Autodesk Inventor part; units mm, degrees
note: some values were not read from the file. Chosen so that the rebuilt part matches the saved one: direction of "Hole2".
(part 7 of 18)
  spline S53 degree 3 poles (-10045.5969, -10030.692) (-10045.5963, -10030.6873) (-10045.5949, -10030.677) (-10045.5853, -10030.6623) (-10045.5707, -10030.6477) (-10045.5504, -10030.6334) (-10045.5248, -10030.6195) (-10045.482, -10030.6008) (-10045.433, -10030.585) (-10045.3785, -10030.5714) (-10045.3141, -10030.5581) (-10045.2258, -10030.5447) (-10045.1146, -10030.5354) (-10045, -10030.532) (-10044.8854, -10030.5354) (-10044.7742, -10030.5447) (-10044.6859, -10030.5581) (-10044.6215, -10030.5714) (-10044.567, -10030.585) (-10044.518, -10030.6008) (-10044.4752, -10030.6195) (-10044.4496, -10030.6334) (-10044.4293, -10030.6477) (-10044.4147, -10030.6623) (-10044.4051, -10030.677) (-10044.4037, -10030.6873) (-10044.4031, -10030.692) knots 0 0 0 0 0.011067 0.024078 0.039928 0.05914 0.081934 0.10802 0.168059 0.202015 0.239296 0.321668 0.410563 0.5 0.589437 0.678332 0.760704 0.797985 0.831941 0.89198 0.918066 0.94086 0.960072 0.975922 0.988933 1 1 1 1
  spline S54 degree 3 poles (-10044.4031, -10030.692) (-10044.4037, -10030.6967) (-10044.405, -10030.7067) (-10044.4147, -10030.7206) (-10044.4293, -10030.7339) (-10044.4497, -10030.7464) (-10044.4753, -10030.758) (-10044.5182, -10030.7731) (-10044.5672, -10030.7852) (-10044.6216, -10030.7953) (-10044.6861, -10030.8049) (-10044.7744, -10030.8142) (-10044.8855, -10030.8205) (-10045, -10030.8227) (-10045.1145, -10030.8205) (-10045.2256, -10030.8142) (-10045.3139, -10030.8049) (-10045.3784, -10030.7953) (-10045.4328, -10030.7852) (-10045.4818, -10030.7731) (-10045.5247, -10030.758) (-10045.5503, -10030.7464) (-10045.5707, -10030.7339) (-10045.5853, -10030.7206) (-10045.595, -10030.7067) (-10045.5963, -10030.6967) (-10045.5969, -10030.692) knots 0 0 0 0 0.010997 0.023628 0.038954 0.057614 0.079908 0.105595 0.165209 0.199149 0.236543 0.319515 0.409403 0.5 0.590597 0.680485 0.763457 0.800851 0.834791 0.894405 0.920092 0.942386 0.961046 0.976372 0.989003 1 1 1 1
  spline S55 degree 3 poles (-10044.4031, -10007.502) (-10044.4037, -10007.5067) (-10044.4051, -10007.517) (-10044.4147, -10007.5317) (-10044.4293, -10007.5463) (-10044.4496, -10007.5606) (-10044.4752, -10007.5745) (-10044.518, -10007.5931) (-10044.567, -10007.6089) (-10044.6215, -10007.6226) (-10044.6859, -10007.6359) (-10044.7742, -10007.6492) (-10044.8854, -10007.6586) (-10045, -10007.6619) (-10045.1146, -10007.6586) (-10045.2258, -10007.6492) (-10045.3141, -10007.6359) (-10045.3785, -10007.6226) (-10045.433, -10007.6089) (-10045.482, -10007.5931) (-10045.5248, -10007.5745) (-10045.5504, -10007.5606) (-10045.5707, -10007.5463) (-10045.5853, -10007.5317) (-10045.5949, -10007.517) (-10045.5963, -10007.5067) (-10045.5969, -10007.502) knots 0 0 0 0 0.011067 0.024078 0.039928 0.05914 0.081934 0.10802 0.168059 0.202015 0.239296 0.321668 0.410563 0.5 0.589437 0.678332 0.760704 0.797985 0.831941 0.89198 0.918066 0.94086 0.960072 0.975922 0.988933 1 1 1 1
  spline S56 degree 3 poles (-10045.5969, -10007.502) (-10045.5963, -10007.4973) (-10045.595, -10007.4873) (-10045.5853, -10007.4734) (-10045.5707, -10007.4601) (-10045.5503, -10007.4476) (-10045.5247, -10007.436) (-10045.4818, -10007.4208) (-10045.4328, -10007.4087) (-10045.3784, -10007.3987) (-10045.3139, -10007.3891) (-10045.2256, -10007.3798) (-10045.1145, -10007.3735) (-10045, -10007.3713) (-10044.8855, -10007.3735) (-10044.7744, -10007.3798) (-10044.6861, -10007.3891) (-10044.6216, -10007.3987) (-10044.5672, -10007.4087) (-10044.5182, -10007.4208) (-10044.4753, -10007.436) (-10044.4497, -10007.4476) (-10044.4293, -10007.4601) (-10044.4147, -10007.4734) (-10044.405, -10007.4873) (-10044.4037, -10007.4973) (-10044.4031, -10007.502) knots 0 0 0 0 0.010997 0.023628 0.038954 0.057614 0.079908 0.105595 0.165209 0.199149 0.236543 0.319515 0.409403 0.5 0.590597 0.680485 0.763457 0.800851 0.834791 0.894405 0.920092 0.942386 0.961046 0.976372 0.989003 1 1 1 1
  line L1792 (-10042.592, -10023.3102) -> (-10042.5, -10023.3102)
  line L1793 (-10042.5, -10028.2512) -> (-10043.1, -10028.2512)
  line L1794 (-10042.5, -10023.3102) -> (-10042.5, -10028.2512)
  line L1795 (-10042.5, -10014.8837) -> (-10042.592, -10014.8837)
  line L1796 (-10042.5, -10009.9428) -> (-10042.5, -10014.8837)
  line L1797 (-10043.1, -10009.9428) -> (-10042.5, -10009.9428)
  line L1798 (-10043.1, -10023.097) -> (-10043.1, -10028.2512)
  line L1799 (-10043.1, -10009.9428) -> (-10043.1, -10015.097)
  line L1800 (-10042.5, -10007.147) -> (-10042.5, -10009.9428)
  line L1801 (-10042.5, -10028.2512) -> (-10042.5, -10031.047)
  line L1802 (-10047.5, -10015.097) -> (-10047.5, -10007.147)
  line L1803 (-10047.5, -10031.047) -> (-10047.5, -10023.097)
  line L1804 (-10042.5, -10031.047) -> (-10047.5, -10031.047)
  line L1805 (-10042.5, -10007.147) -> (-10047.5, -10007.147)
  line L1806 (-10042.5, -10014.8837) -> (-10042.5, -10015.1936)
  line L1807 (-10042.5, -10015.1936) -> (-10042.592, -10015.1936)
  line L1808 (-10042.5, -10015.1936) -> (-10042.5, -10023.3102)
  line L1809 (-10057.5, -10028.1794) -> (-10057.5, -10022.4221)
  line L1810 (-10057.5, -10015.7719) -> (-10057.5, -10010.0146)
  line L1811 (-10057.5, -10008.4468) -> (-10057.5, -10007.8837)
  line L1812 (-10057.5, -10030.3103) -> (-10057.5, -10029.7472)
  line L1813 (-10047.5, -10007.8837) -> (-10057.5, -10007.8837)
  line L1814 (-10057.5, -10030.3103) -> (-10047.5, -10030.3103)
  spline S57 degree 3 poles (-10050.101, -10027.8648) (-10050.2112, -10027.8645) (-10050.4351, -10027.8611) (-10050.7676, -10027.843) (-10051.0408, -10027.8129) (-10051.2301, -10027.7795) (-10051.3223, -10027.7451) (-10051.3848, -10027.7216) (-10051.3872, -10027.6724) (-10051.3472, -10027.6448) (-10051.2666, -10027.61) (-10051.0804, -10027.5729) (-10050.8071, -10027.5414) (-10050.4756, -10027.5234) (-10050.1423, -10027.519) (-10049.8093, -10027.5266) (-10049.4755, -10027.5466) (-10049.2034, -10027.5785) (-10049.0137, -10027.6143) (-10048.9225, -10027.6467) (-10048.8568, -10027.6705) (-10048.8566, -10027.7199) (-10048.8981, -10027.7462) (-10048.9787, -10027.777) (-10049.1645, -10027.8141) (-10049.4369, -10027.8433) (-10049.7691, -10027.8609) (-10049.9917, -10027.865) (-10050.101, -10027.8648) knots 0 0 0 0 0.063707 0.129495 0.191912 0.223688 0.23829 0.25135 0.256604 0.263018 0.277149 0.308538 0.37104 0.436878 0.500023 0.563695 0.629383 0.692836 0.723161 0.738573 0.75181 0.756962 0.76326 0.777952 0.808043 0.871314 0.936843 1 1 1 1
  spline S58 degree 3 poles (-10050.1826, -10030.061) (-10050.4053, -10030.0603) (-10050.7291, -10030.05) (-10051.1255, -10030.0499) (-10051.2836, -10030.0122) (-10051.3774, -10030.0214) (-10051.3875, -10029.9848) (-10051.307, -10029.9741) (-10051.2197, -10029.9555) (-10050.9994, -10029.9405) (-10050.7296, -10029.927) (-10050.3957, -10029.9197) (-10049.9493, -10029.9156) (-10049.5164, -10029.9313) (-10049.1193, -10029.9348) (-10048.9604, -10029.9745) (-10048.8659, -10029.9652) (-10048.8554, -10030.0025) (-10048.9378, -10030.0112) (-10049.0249, -10030.0292) (-10049.246, -10030.0414) (-10049.6233, -10030.0575) (-10049.9596, -10030.0616) (-10050.1826, -10030.061) knots 0 0 0 0 0.131392 0.195062 0.224866 0.236537 0.238771 0.243638 0.272647 0.302988 0.368078 0.435032 0.499113 0.631038 0.694715 0.724747 0.73665 0.738894 0.743873 0.773079 0.803452 0.868455 1 1 1 1
  spline S59 degree 3 poles (-10050.1826, -10010.6731) (-10050.2929, -10010.6727) (-10050.5175, -10010.6697) (-10050.8464, -10010.6478) (-10051.127, -10010.6184) (-10051.2936, -10010.571) (-10051.3855, -10010.5349) (-10051.3867, -10010.4859) (-10051.3246, -10010.4425) (-10051.2136, -10010.412) (-10051.0014, -10010.3752) (-10050.7253, -10010.348) (-10050.394, -10010.3316) (-10050.0607, -10010.3274) (-10049.7273, -10010.3345) (-10049.3981, -10010.354) (-10049.1186, -10010.3846) (-10048.951, -10010.4283) (-10048.8591, -10010.4605) (-10048.8553, -10010.51) (-10048.9209, -10010.5537) (-10049.03, -10010.5814) (-10049.2424, -10010.6228) (-10049.5173, -10010.6499) (-10049.8505, -10010.669) (-10050.0733, -10010.6734) (-10050.1826, -10010.6731) knots 0 0 0 0 0.063774 0.129476 0.191917 0.222516 0.235727 0.240982 0.247121 0.27643 0.308417 0.371002 0.43691 0.500019 0.563738 0.62925 0.691939 0.722123 0.735387 0.74054 0.746943 0.777028 0.807219 0.871188 0.93687 1 1 1 1
  line L1815 (-10057.5, -10010.0146) -> (-10057.5, -10008.4468)
  line L1816 (-10057.5, -10029.7472) -> (-10057.5, -10028.1794)
  spline S60 degree 3 poles (-10050.101, -10008.2758) (-10050.3249, -10008.2751) (-10050.6589, -10008.2732) (-10051.0379, -10008.2488) (-10051.2309, -10008.2402) (-10051.3162, -10008.2166) (-10051.382, -10008.2231) (-10051.3853, -10008.1857) (-10051.34, -10008.1823) (-10051.2677, -10008.1628) (-10051.076, -10008.154) (-10050.8073, -10008.1395) (-10050.475, -10008.134) (-10050.0295, -10008.1322) (-10049.5838, -10008.1356) (-10049.2069, -10008.1566) (-10049.0122, -10008.164) (-10048.9298, -10008.1856) (-10048.8582, -10008.1781) (-10048.8591, -10008.2157) (-10048.9046, -10008.2188) (-10048.9776, -10008.2383) (-10049.1684, -10008.2498) (-10049.5444, -10008.2725) (-10049.8785, -10008.2765) (-10050.101, -10008.2758) knots 0 0 0 0 0.132092 0.195475 0.227359 0.241584 0.252969 0.255186 0.260256 0.27356 0.304855 0.368241 0.435353 0.499807 0.631725 0.696074 0.726444 0.741485 0.752997 0.755195 0.760334 0.774394 0.8045 0.86873 1 1 1 1
  line L1817 (-10055.03, -10015.097) -> (-10062.35, -10017.097)
  line L1818 (-10062.35, -10021.097) -> (-10055.03, -10023.097)
  line L1819 (-10043.608, -10015.097) -> (-10055.03, -10015.097)
  line L1820 (-10043.608, -10023.097) -> (-10055.03, -10023.097)
  line L1821 (-10062.35, -10017.097) -> (-10062.35, -10021.097)
  line L1822 (-10043.608, -10015.097) -> (-10042.592, -10015.097)
  line L1823 (-10043.608, -10023.097) -> (-10042.592, -10023.097)
  line L1824 (-10042.592, -10015.097) -> (-10042.592, -10023.097)
  line L1825 (-10042.592, -10027.222) -> (-10042.592, -10027.3968)
  line L1826 (-10043.1, -10027.222) -> (-10042.592, -10027.222)
  line L1827 (-10042.592, -10023.5196) -> (-10042.592, -10027.222)
  line L1828 (-10042.592, -10023.5196) -> (-10042.592, -10023.097)
  line L1829 (-10042.592, -10015.097) -> (-10042.592, -10014.6744)
  line L1830 (-10042.592, -10010.972) -> (-10042.592, -10014.6744)
  line L1831 (-10043.1, -10010.972) -> (-10042.592, -10010.972)
  line L1832 (-10042.592, -10010.7972) -> (-10042.592, -10010.972)
  line L1833 (-10043.1, -10027.3968) -> (-10042.592, -10027.3968)
  line L1834 (-10043.1, -10010.7972) -> (-10042.592, -10010.7972)
  line L1835 (-10039.5, -10030.097) -> (-10039.5, -10008.097)
  line L1836 (-10006.5, -10030.097) -> (-10006.5, -10008.097)
  line L1837 (-10006.5, -10030.097) -> (-10039.5, -10030.097)
  line L1838 (-10006.5, -10008.097) -> (-10039.5, -10008.097)
  line L1839 (-10039.5, -10028.4955) -> (-10042.5, -10028.4955)
  line L1840 (-10039.5, -10026.3955) -> (-10042.5, -10026.3955)
  line L1841 (-10039.5, -10020.147) -> (-10042.5, -10020.147)
  line L1842 (-10039.5, -10018.047) -> (-10042.5, -10018.047)
  line L1843 (-10039.5, -10011.7985) -> (-10042.5, -10011.7985)
  line L1844 (-10039.5, -10009.6985) -> (-10042.5, -10009.6985)
  point P0 (-10071.5736, -10018.3821)
  point P1 (-10089.4145, -10025.2382)
  point P2 (-10089.4707, -10025.1054)
  point P3 (-10089.5241, -10024.9747)
  point P4 (-10089.5748, -10024.8458)
  point P5 (-10089.668, -10024.5932)
  point P6 (-10089.71, -10026.541)
  point P7 (-10089.7079, -10026.5802)
  point P8 (-10089.7068, -10026.6181)
  point P9 (-10089.7067, -10026.6545)
  point P10 (-10089.7078, -10026.6891)
  point P11 (-10089.7099, -10026.7219)
  point P12 (-10089.7131, -10026.7527)
  point P13 (-10089.7174, -10026.7816)
  point P14 (-10089.7226, -10026.8085)
  point P15 (-10089.7286, -10026.8333)
  point P16 (-10089.7356, -10026.8561)
  point P17 (-10089.7434, -10026.8767)
  point P18 (-10089.7519, -10026.8952)
  point P19 (-10089.7614, -10026.912)
  point P20 (-10089.7719, -10026.9273)
  point P21 (-10089.5643, -10022.119)
  point P22 (-10089.6337, -10021.9928)
  point P23 (-10089.7001, -10021.8683)
  point P24 (-10089.7635, -10021.7454)
  point P25 (-10089.8819, -10021.5039)
  point P26 (-10089.8819, -10016.6901)
  point P27 (-10089.7635, -10016.4486)
  point P28 (-10089.7001, -10016.3257)
  point P29 (-10089.6337, -10016.2012)
  point P30 (-10089.5643, -10016.075)
  point P31 (-10089.668, -10013.6008)
  point P32 (-10089.5748, -10013.3482)
  point P33 (-10089.5241, -10013.2193)
  point P34 (-10089.4707, -10013.0885)
  point P35 (-10089.4145, -10012.9558)
  point P36 (-10089.7719, -10011.2677)
  point P37 (-10089.7611, -10011.2837)
  point P38 (-10089.7512, -10011.3016)
  point P39 (-10089.7423, -10011.3212)
  point P40 (-10089.7344, -10011.3427)
  point P41 (-10089.7274, -10011.3659)
  point P42 (-10089.7214, -10011.3908)
  point P43 (-10089.7164, -10011.4174)
  point P44 (-10089.7125, -10011.4458)
  point P45 (-10089.7096, -10011.4759)
  point P46 (-10089.7077, -10011.5079)
  point P47 (-10089.7068, -10011.5416)
  point P48 (-10089.707, -10011.5772)
  point P49 (-10089.7081, -10011.6144)
  point P50 (-10089.7102, -10011.6532)
  point P51 (-10091.3425, -10024.7667)
  point P52 (-10091.4, -10024.6345)
  point P53 (-10091.4547, -10024.5043)
  point P54 (-10091.5066, -10024.3759)
  point P55 (-10091.6023, -10024.1243)
  point P56 (-10091.7673, -10025.3691)
  point P57 (-10091.7263, -10025.5187)
  point P58 (-10091.6914, -10025.6621)
  point P59 (-10091.663, -10025.7981)
  point P60 (-10091.6416, -10025.9259)
  point P61 (-10091.6273, -10026.0484)
  point P62 (-10091.6212, -10026.1625)
  point P63 (-10091.6215, -10026.2148)
  point P64 (-10091.6244, -10026.263)
  point P65 (-10091.6295, -10026.307)
  point P66 (-10091.6368, -10026.3467)
  point P67 (-10091.6462, -10026.3819)
  point P68 (-10091.6573, -10026.4125)
  point P69 (-10091.6855, -10026.4616)
  point P70 (-10091.7224, -10026.4967)
  point P71 (-10091.7672, -10026.5165)
  point P72 (-10091.8189, -10026.5203)
  point P73 (-10091.8754, -10026.5098)
  point P74 (-10091.4781, -10022.119)
  point P75 (-10091.5475, -10021.9928)
  point P76 (-10091.6139, -10021.8683)
  point P77 (-10091.6774, -10021.7454)
  point P78 (-10091.7959, -10021.5039)
  point P79 (-10091.7959, -10016.6901)
  point P80 (-10091.6774, -10016.4486)
  point P81 (-10091.6139, -10016.3257)
  point P82 (-10091.5475, -10016.2012)
  point P83 (-10091.4781, -10016.075)
  point P84 (-10091.7589, -10022.7293)
  point P85 (-10091.7079, -10022.8468)
  point P86 (-10091.6604, -10022.9609)
  point P87 (-10091.6166, -10023.071)
  point P88 (-10091.5769, -10023.1768)
  point P89 (-10091.5414, -10023.2776)
  point P90 (-10091.5098, -10023.3753)
  point P91 (-10091.4824, -10023.4695)
  point P92 (-10091.4603, -10023.5573)
  point P93 (-10091.4446, -10023.6364)
  point P94 (-10091.4354, -10023.7052)
  point P95 (-10091.4324, -10023.7633)
  point P96 (-10091.4352, -10023.8101)
  point P97 (-10091.4439, -10023.8482)
  point P98 (-10091.4584, -10023.8776)
  point P99 (-10091.4589, -10014.3159)
  point P100 (-10091.4446, -10014.3449)
  point P101 (-10091.4359, -10014.3831)
  point P102 (-10091.4327, -10014.4302)
  point P103 (-10091.4352, -10014.4861)
  point P104 (-10091.4434, -10014.5504)
  point P105 (-10091.4575, -10014.6236)
  point P106 (-10091.4774, -10014.7055)
  point P107 (-10091.5029, -10014.7955)
  point P108 (-10091.5337, -10014.8928)
  point P109 (-10091.5695, -10014.9967)
  point P110 (-10091.6103, -10015.1064)
  point P111 (-10091.6555, -10015.2212)
  point P112 (-10091.7048, -10015.34)
  point P113 (-10091.6023, -10014.0697)
  point P114 (-10091.5066, -10013.818)
  point P115 (-10091.4547, -10013.6897)
  point P116 (-10091.4, -10013.5594)
  point P117 (-10091.3425, -10013.4273)
  point P118 (-10091.8739, -10011.6836)
  point P119 (-10091.8177, -10011.6735)
  point P120 (-10091.7673, -10011.6775)
  point P121 (-10091.7235, -10011.6967)
  point P122 (-10091.687, -10011.7313)
  point P123 (-10091.6582, -10011.7809)
  point P124 (-10091.6374, -10011.8451)
  point P125 (-10091.625, -10011.9234)
  point P126 (-10091.6212, -10012.0163)
  point P127 (-10091.6257, -10012.1235)
  point P128 (-10091.6385, -10012.2435)
  point P129 (-10091.6593, -10012.3747)
  point P130 (-10091.6878, -10012.5159)
  point P131 (-10091.7237, -10012.6653)
  point P132 (-10091.7661, -10012.8207)
  point P133 (-10070.533, -10008.749)
  point P134 (-10070.5501, -10008.7522)
  point P135 (-10070.5668, -10008.7563)
  point P136 (-10070.583, -10008.7615)
  point P137 (-10070.5987, -10008.7675)
  point P138 (-10070.6138, -10008.7744)
  point P139 (-10070.6283, -10008.7822)
  point P140 (-10070.6421, -10008.7907)
  point P141 (-10070.6551, -10008.8001)
  point P142 (-10070.6673, -10008.8101)
  point P143 (-10070.6786, -10008.8209)
  point P144 (-10070.689, -10008.8323)
  point P145 (-10070.6984, -10008.8443)
  point P146 (-10070.7067, -10008.8568)
  point P147 (-10070.7139, -10008.87)
  point P148 (-10070.7067, -10009.0292)
  point P149 (-10070.6997, -10009.0407)
  point P150 (-10070.6918, -10009.0517)
  point P151 (-10070.6833, -10009.0623)
  point P152 (-10070.6741, -10009.0724)
  point P153 (-10070.6642, -10009.082)
  point P154 (-10070.6537, -10009.091)
  point P155 (-10070.6427, -10009.0995)
  point P156 (-10070.6311, -10009.1075)
  point P157 (-10070.6191, -10009.1148)
  point P158 (-10070.6066, -10009.1215)
  point P159 (-10070.5938, -10009.1276)
  point P160 (-10070.5806, -10009.133)
  point P161 (-10070.5671, -10009.1377)
  point P162 (-10070.5534, -10009.1417)
  point P163 (-10070.5608, -10009.1684)
  point P164 (-10070.5743, -10009.1636)
  point P165 (-10070.5875, -10009.158)
  point P166 (-10070.6003, -10009.1514)
  point P167 (-10070.6127, -10009.144)
  point P168 (-10070.6248, -10009.1358)
  point P169 (-10070.6364, -10009.1269)
  point P170 (-10070.6475, -10009.1173)
  point P171 (-10070.6581, -10009.107)
  point P172 (-10070.6682, -10009.0962)
  point P173 (-10070.6778, -10009.0848)
  point P174 (-10070.6868, -10009.0728)
  point P175 (-10070.6951, -10009.0604)
  point P176 (-10070.7029, -10009.0476)
  point P177 (-10070.7099, -10009.0344)
  point P178 (-10070.737, -10008.8939)
  point P179 (-10070.7333, -10008.8725)
  point P180 (-10070.7274, -10008.8517)
  point P181 (-10070.7195, -10008.832)
  point P182 (-10070.7097, -10008.8138)
  point P183 (-10070.6981, -10008.7969)
  point P184 (-10070.685, -10008.7815)
  point P185 (-10070.6705, -10008.7675)
  point P186 (-10070.6546, -10008.7548)
  point P187 (-10070.6376, -10008.7436)
  point P188 (-10070.6196, -10008.7337)
  point P189 (-10070.6007, -10008.7252)
  point P190 (-10070.5811, -10008.7181)
  point P191 (-10070.5608, -10008.7123)
  point P192 (-10070.5401, -10008.7079)
  point P193 (-10070.3883, -10008.7119)
  point P194 (-10070.3706, -10008.7176)
  point P195 (-10070.3539, -10008.7248)
  point P196 (-10070.3382, -10008.7334)
  point P197 (-10070.3237, -10008.7435)
  point P198 (-10070.3103, -10008.7548)
  point P199 (-10070.2981, -10008.7674)
sketch "Sketch2" plane through (0, 0, 0) normal (1, 0, 0) x (0, 1, 0)
  line L0 (0, -156.7871) -> (0, 91.8442) projected
  line L1 (-13, 0) -> (12, 0)
  line L2 (-13, 0) -> (-13.762, 0)
  line L3 (-11, 25) -> (0, 25)
  line L4 (-11, 23.984) -> (-11, 25)
  line L5 (-8.5, 10) -> (8.5, 10)
  line L6 (8.5, 10) -> (8.5, 0)
  line L7 (8.5, 0) -> (-8.5, 0)
  line L8 (-8.5, 0) -> (-8.5, 10)
  line L9 (-12, 5) -> (12, 5)
  line L10 (12, 5) -> (12, 0)
  line L11 (12, 0) -> (-12, 0)
  line L12 (-12, 0) -> (-12, 5)
  line L13 (-7.484, 10) -> (-7.484, 0)
  line L14 (-10.984, 5) -> (-10.984, 0)
  spline S0 degree 4 poles (-11, 23.984) (-11, 20.7131) (-6.8945, 12.8732) (-7.9989, 10.3689) (-11.1719, 5.7207) (-13.5566, 3.5083) (-13.762, 1.3879) (-13.762, 0) knots 0 0 0 0 0 0.403232 0.585845 0.725536 1 1 1 1 1
  spline S1 degree 4 poles (-10.4574, 23.2133) (-10.1643, 18.8628) (-2.9804, 8.5508) (-10.8366, 7.0695) (-13, 2.344) (-13, 0) knots 0 0 0 0 0 0.540079 1 1 1 1 1
  line L15 (-10.2082, 7.2459) -> (-13.7918, 2.7541) construction
  arc A0 (-10.476, 6.7064) -> (-13.3253, 3.1351) centre (4.0982, -7.8437) ccw construction
  line L16 (-7.7665, 11.7153) -> (-9.2335, 8.2847) construction
  arc A1 (-9.2262, 8.7305) -> (-8.0838, 11.402) centre (-14.3346, 12.4949) ccw construction
  line L17 (0, 23.984) -> (0, 25)
  line L18 (-13, 0) -> (-13, -15)
  line L19 (-13.762, 0) -> (-13.762, -15)
  arc A2 (-9.484, 23.984) -> (-10.4574, 23.2133) centre (-9.484, 22.984) ccw
  line L20 (-10.6483, 26.0474) -> (-10.2664, 20.3792) construction
  arc A3 (-10.272, 25.3991) -> (-9.9805, 21.0721) centre (-3.2242, 23.7006) ccw construction
  line L21 (0, 23.984) -> (-9.484, 23.984)
  line L22 (-10.984, 23.984) -> (-11, 23.984)
  line L23 (-13.762, -15) -> (-13, -15)
  circle A4 centre (-10, 24) radius 1
  point P0 (0, 0)
  point P1 (0, 0)
  point P2 (0, 10)
  dimension "d16" = 25
  dimension "d17" = 17
  dimension "d18" = 10
  dimension "d19" = 24
  dimension "d20" = 5
  dimension "d22" = 1.016
  dimension "d23" = 1.016
  dimension "d25" = 2
  dimension "d26" = 15
  dimension "d27" = 0.762
  dimension "d28" = 13
  dimension "d91" = 11
  dimension "d92" = 2
  constraints: 46 end point, 10 parallel, 9 midpoint, 7 point on line, 5 centre point, 5 horizontal, 5 point on circle, 4 coincident, 4 perpendicular, 4 tangent, 3 vertical, 2 vertical alignment, 15 other
  measures "d16" distance between parallel lines of L1 L3
  measures "d17" distance between parallel lines of L6 L8
  measures "d18" distance between parallel lines of L7 L5
  measures "d19" distance between parallel lines of L10 L12
  measures "d20" distance between parallel lines of L11 L9
  measures "d22" distance between parallel lines of L13 L8
  measures "d23" distance between parallel lines of L14 L12
  measures "d25" diameter of A2
  measures "d26" distance of L19.end L2.end
  measures "d27" distance of L1.start L2.end
  measures "d28" distance of point (0, 0) L1.start
  measures "d91" distance of L3.end L3.start
  measures "d92" diameter of A4
revolve "Revolution1" [suppressed]
revolve "Mid Thick" add sketch "Sketch2" angle 360 about axis through (0, 0, -10) along (0, 0, 1) contours L2 L18 L23 L19
sketch "Sketch4" plane through (0, 0, 0) normal (1, 0, 0) x (0, 1, 0)
  line L0 (13.762, -15) -> (-13.762, -15) projected
  line L1 (0, -156.7871) -> (0, 91.8442) projected
  line L2 (-12, -15) -> (12, -15)
  line L3 (12, -15) -> (12, -29.9769)
  line L4 (12, -29.9769) -> (-12, -29.9769)
  line L5 (-12, -29.9769) -> (-12, -15)
  line L6 (-12, -29.9769) -> (-13.016, -29.9769)
  line L7 (-12, -25) -> (-12, -29.9769)
  line L8 (-13.762, -15) -> (-13.762, 0) projected
  line L9 (-13, 0) -> (-13, -15) projected
  spline S0 degree 4 poles (-13, -15) (-13, -16.8784) (-13, -20.6351) (-12, -24.3418) (-12, -28.0985) (-12, -29.9769) knots 0 0 0 0 0 0.5 1 1 1 1 1
  line L10 (-13.016, -29.9769) -> (-13.016, -27.4885)
  spline S1 degree 4 poles (-13.762, -15) (-13.762, -16.8756) (-13.762, -20.6268) (-13.016, -24.3501) (-13.016, -28.1013) (-13.016, -29.9769) knots 0 0 0 0 0 0.5 1 1 1 1 1
  line L11 (-13.762, -15) -> (-13, -15)
  point P0 (0, 0)
  point P1 (0, -15)
  point P2 (0, -15)
  dimension "d34" = 24
  dimension "d37" = 1.016
  constraints: 16 end point, 4 vertical, 3 parallel, 2 horizontal, 2 midpoint, 1 coincident, 1 collinear, 1 perpendicular, 1 point on line, 4 other
  measures "d34" distance between parallel lines of L3 L5
  measures "d37" distance of L4.end L6.end
revolve "Mid Tran" add sketch "Sketch4" angle 360 about axis through (0, 0, -10) along (0, 0, 1) contours S0 L6 S1 L0
sketch "Sketch5" plane through (0, 0, 0) normal (1, 0, 0) x (0, 1, 0)
  line L0 (13.016, -29.9769) -> (-13.016, -29.9769) projected
  line L1 (12, -29.9769) -> (-12, -29.9769) projected
  line L2 (0, -156.7871) -> (0, 91.8442) projected
  line L3 (-12, -29.9769) -> (14, -29.9769)
  line L4 (14, -29.9769) -> (14, -64.9769)
  line L5 (14, -64.9769) -> (-12, -64.9769)
  line L6 (-12, -64.9769) -> (-12, -29.9769)
  line L7 (-12, -29.9769) -> (-13.016, -29.9769)
  line L8 (-12, -64.9769) -> (-13.016, -64.9769)
  line L9 (-13.016, -64.9769) -> (-13.016, -29.9769)
  point P0 (0, 0)
  dimension "d39" = 26
  dimension "d40" = 1.016
  dimension "d41" = 35
  constraints: 14 end point, 3 parallel, 2 perpendicular, 1 horizontal
  measures "d39" distance between parallel lines of L4 L6
  measures "d40" distance of L5.end L8.end
  measures "d41" distance between parallel lines of L5 L0
revolve "Thin" add sketch "Sketch5" angle 360 about axis through (0, 0, -10) along (0, 0, 1) contours L6 L8 L9 L0
sketch "Sketch7" plane through (0, 0, -64.9769) normal (0, 0, -1) x (-1, 0, 0)
  circle A0 centre (0, 0) radius 13.016 projected
  circle A1 centre (0, 0) radius 12 projected
  circle A2 centre (0, 0) radius 13.016
  constraints: 1 centre point, 1 coincident, 1 concentric
ref_plane "Work Plane5" through (0, 0, -64.9769) normal (0, 0, 1) x (1, 0, 0)
extrude "Extrusion1" add sketch "Sketch7" along normal blind 4 contours A0 | A1
sketch "Sketch8" plane through (0, 0, -68.9769) normal (0, 0, -1) x (-1, 0, 0)
  circle A0 centre (0, 0) radius 13.016 projected
  line L0 (7.5823, 2.074) -> (6.4276, 4.074)
  line L1 (6.4276, 4.074) -> (7.5823, 6.074)
  line L2 (7.5823, 6.074) -> (9.8917, 6.074)
  line L3 (9.8917, 6.074) -> (11.0464, 4.074)
  line L4 (11.0464, 4.074) -> (9.8917, 2.074)
  line L5 (9.8917, 2.074) -> (7.5823, 2.074)
  line L6 (0, -149.7222) -> (0, 130.9275) projected
  line L7 (-9.5037, 6.82) -> (-7.1943, 6.82)
  line L8 (-7.1943, 6.82) -> (-6.0396, 4.82)
  line L9 (-6.0396, 4.82) -> (-7.1943, 2.82)
  line L10 (-7.1943, 2.82) -> (-9.5037, 2.82)
  line L11 (-9.5037, 2.82) -> (-10.6584, 4.82)
  line L12 (-10.6584, 4.82) -> (-9.5037, 6.82)
  line L13 (1.1547, -7.494) -> (2.3094, -9.494)
  line L14 (2.3094, -9.494) -> (1.1547, -11.494)
  line L15 (1.1547, -11.494) -> (-1.1547, -11.494)
  line L16 (-1.1547, -11.494) -> (-2.3094, -9.494)
  line L17 (-2.3094, -9.494) -> (-1.1547, -7.494)
  line L18 (-1.1547, -7.494) -> (1.1547, -7.494)
  point P0 (8.737, 4.074)
  point P1 (-8.349, 4.82)
  point P2 (0, -9.494)
  point P3 (8.737, 4.074)
  dimension "d45" = 4.074
  dimension "d46" = 8.737
  dimension "d47" = 4.82
  dimension "d48" = 8.349
  dimension "d49" = 9.494
  dimension "d51" = 4
  dimension "d52" = 4
  dimension "d53" = 4
  constraints: 36 end point, 1 coincident, 1 other
  measures "d45" vertical distance of point (8.737, 4.074) A0.centre
  measures "d46" horizontal distance of point (8.737, 4.074) A0.centre
  measures "d47" vertical distance of point (-8.349, 4.82) A0.centre
  measures "d48" horizontal distance of A0.centre point (-8.349, 4.82)
  measures "d49" distance of point (0, -9.494) A0.centre
  measures "d51" distance between parallel lines of L0 L3
  measures "d52" distance between parallel lines of L7 L10
  measures "d53" distance between parallel lines of L13 L16
hole "Hole1" at (-8.737, 4.074, -68.9769) at (8.349, 4.82, -68.9769) at (0, -9.494, -68.9769) at (-8.737, 4.074, -68.9769) direction (0, 0, 1) diameter 1.778 depth 4 clearance for "Flat Head Machine Screw (82)" size "#0" standard "Ansi Unified Screw Threads"
sketch "Sketch9" plane through (0, 0, 0) normal (1, 0, 0) x (0, 1, 0)
  line L0 (-13.016, -68.9769) -> (-13.016, -29.9769) projected
  line L1 (13.016, -68.9769) -> (-13.016, -68.9769) projected
  line L2 (0, -156.7871) -> (0, 91.8442) projected
  line L3 (-8, -68.9769) -> (0, -68.9769)
  line L4 (0, -68.9769) -> (0, -88.9769)
  line L5 (0, -88.9769) -> (-5, -88.9769)
  spline S0 degree 3 poles (-13.016, -68.9769) (-13.016, -76.4169) (-13.016, -83.8568) (-5, -88.9769) knots 0 0 0 0 1 1 1 1
  line L6 (-13.016, -68.9769) -> (-8, -68.9769)
  point P0 (0, 0)
  point P1 (-4, -68.9769)
  dimension "d68" = 20
  dimension "d102" = 5
  constraints: 8 end point, 2 midpoint, 1 coincident, 1 horizontal, 1 horizontal alignment, 1 parallel, 1 perpendicular, 1 vertical, 2 other
  measures "d68" distance between parallel lines of L5 L3
  measures "d102" distance of L4.end L5.end
revolve "Revolution6" add sketch "Sketch9" angle 360 about axis through (0, 0, -10) along (0, 0, 1)
ref_plane "Work Plane6" through (0, 0, -67.4769) normal (0, 0, 1) x (1, 0, 0)
sketch "Sketch11" plane through (0, 0, -67.4769) normal (0, 0, 1) x (1, 0, 0)
  circle A0 centre (-8.737, 4.074) radius 0.889 projected
  circle A1 centre (8.349, 4.82) radius 0.889 projected
  circle A2 centre (0, -9.494) radius 0.889 projected
  line L0 (-9.8917, 2.074) -> (-7.5823, 2.074) projected
  line L1 (-11.0464, 4.074) -> (-9.8917, 2.074) projected
  line L2 (-7.5823, 2.074) -> (-6.4276, 4.074) projected
  line L3 (-9.8917, 6.074) -> (-11.0464, 4.074) projected
  line L4 (-7.5823, 6.074) -> (-9.8917, 6.074) projected
  line L5 (-6.4276, 4.074) -> (-7.5823, 6.074) projected
  line L6 (1.1547, -7.494) -> (-1.1547, -7.494) projected
  line L7 (2.3094, -9.494) -> (1.1547, -7.494) projected
  line L8 (1.1547, -11.494) -> (2.3094, -9.494) projected
  line L9 (-1.1547, -11.494) -> (1.1547, -11.494) projected
  line L10 (-2.3094, -9.494) -> (-1.1547, -11.494) projected
  line L11 (-1.1547, -7.494) -> (-2.3094, -9.494) projected
  line L12 (7.1943, 6.82) -> (6.0396, 4.82) projected
  line L13 (9.5037, 6.82) -> (7.1943, 6.82) projected
  line L14 (10.6584, 4.82) -> (9.5037, 6.82) projected
  line L15 (9.5037, 2.82) -> (10.6584, 4.82) projected
  line L16 (7.1943, 2.82) -> (9.5037, 2.82) projected
  line L17 (6.0396, 4.82) -> (7.1943, 2.82) projected
  point P0 (0, 0)
extrude "Extrusion3" cut sketch "Sketch11" against normal through all contours A0 | A1 | A2 | L1 L3 L4 L5 L2 L0 | L7 L8 L9 L10 L11 L6 | L13 L14 L15 L16 L17 L12
ref_plane "Work Plane7" through (0, 0, -64.9769) normal (0, 0, 1) x (1, 0, 0)
hole "Hole2" at (0, 0, -88.9769) direction (0, 0, 1) diameter 10 depth 24
sketch "Sketch12" plane through (0, 0, 0) normal (1, 0, 0) x (0, 1, 0)
  spline S0 degree 3 poles (67.0407, -110.3407) (67.1817, -110.7544) (67.4681, -111.5946) (67.8445, -112.9006) (68.1655, -114.2768) (68.4036, -115.6894) (68.5535, -117.0906) (68.6289, -118.4389) (68.6542, -119.7414) (68.6542, -120.596) (68.6542, -121.0183) knots 0 0 0 0 0.131107 0.266278 0.407581 0.554823 0.69573 0.830104 0.959816 1.086502 1.086502 1.086502 1.086502
  spline S1 degree 3 poles (65.0407, -106.0362) (65.0407, -106.036) (65.0407, -106.0351) (65.0407, -106.0332) (65.0407, -106.0301) (65.0407, -106.0256) (65.0407, -106.02) (65.0407, -106.013) (65.0407, -106.0048) (65.0407, -105.9954) (65.0407, -105.9848) (65.0407, -105.9729) (65.0407, -105.9598) (65.0407, -105.9455) (65.0407, -105.9301) (65.0407, -105.9134) (65.0407, -105.8957) (65.0407, -105.8834) (65.0407, -105.8771) knots 0 0 0 0 0.003987 0.015957 0.035891 0.063749 0.099497 0.143102 0.194528 0.253743 0.320712 0.395401 0.477746 0.567575 0.664794 0.769325 0.881087 1 1 1 1
  spline S2 degree 3 poles (65.0407, -105.8771) (65.1942, -106.2607) (65.4988, -107.0221) (66.1738, -108.5069) (66.6942, -109.6076) (67.0407, -110.3407) knots 0 0 0 0 0.253343 0.502767 1 1 1 1
  spline S3 degree 3 poles (83.3547, -109.9774) (83.2051, -110.404) (82.9009, -111.2712) (82.4948, -112.6197) (82.1452, -114.044) (81.8839, -115.5078) (81.7188, -116.9595) (81.6357, -118.3541) (81.6079, -119.6997) (81.6078, -120.5822) (81.6078, -121.0183) knots 0 0 0 0 0.135587 0.27568 0.422315 0.575323 0.72143 0.860365 0.994299 1.125132 1.125132 1.125132 1.125132
  line L0 (81.3547, -105.4644) -> (81.3547, -121.0183)
  line L1 (81.6078, -121.0183) -> (81.3547, -121.0183)
  line L2 (81.3547, -121.0183) -> (79.3547, -121.0183)
  spline S4 degree 3 poles (79.3547, -121.0183) (79.3547, -120.136) (79.3547, -118.7916) (79.3547, -116.9633) (79.3547, -115.5153) (79.3547, -114.0544) (79.3547, -112.6299) (79.3547, -111.2799) (79.3547, -110.4048) (79.3547, -109.9771) knots 0 0 0 0 0.264693 0.403339 0.548464 0.699098 0.841605 0.975818 1.104119 1.104119 1.104119 1.104119
  spline S5 degree 3 poles (79.3547, -109.9771) (79.7074, -109.2409) (80.2378, -108.134) (80.8185, -106.821) (81.1331, -106.0532) (81.2805, -105.6615) (81.3547, -105.4644) knots 0 0 0 0 0.495968 0.745691 0.872094 1 1 1 1
  spline S6 degree 3 poles (81.3547, -105.4644) (81.4363, -105.4894) (81.5989, -105.5393) (81.849, -105.5899) (82.1011, -105.6215) (82.3548, -105.6319) (82.6083, -105.6216) (82.8606, -105.59) (83.1105, -105.5394) (83.2732, -105.4895) (83.3547, -105.4646) knots 0 0 0 0 0.125726 0.250746 0.375528 0.500005 0.624584 0.749245 0.874433 1 1 1 1
  spline S7 degree 3 poles (83.3547, -105.4646) (83.3547, -105.8539) (83.3547, -106.6196) (83.3547, -108.1239) (83.3547, -109.2389) (83.3547, -109.9774) knots 0 0 0 0 0.25882 0.509015 1 1 1 1
  line L3 (67.0407, -94.5183) -> (67.0407, -110.3407)
  line L4 (67.0407, -94.5183) -> (69.0407, -94.5183)
  line L5 (69.0407, -94.5183) -> (69.0407, -121.0183)
  line L6 (65.0407, -94.5183) -> (65.0407, -105.8771)
  line L7 (65.0407, -94.5183) -> (67.0407, -94.5183)
  line L8 (79.3547, -94.5183) -> (79.3547, -109.9771)
  line L9 (79.3547, -94.5183) -> (81.3547, -94.5183)
  line L10 (81.3547, -94.5183) -> (81.3547, -105.4644)
  line L11 (81.3547, -94.5183) -> (83.3547, -94.5183)
  line L12 (83.3547, -94.5183) -> (83.3547, -105.4646)
  line L13 (78.6087, -94.5183) -> (78.6087, -121.0183)
  line L14 (78.6087, -94.5183) -> (79.3547, -94.5183)
  line L15 (80.6087, -94.5183) -> (80.6087, -121.0183)
  line L16 (82.6087, -94.5183) -> (82.6087, -110.4853)
  spline S8 degree 3 poles (80.9874, -121.0183) (80.9875, -120.6017) (80.9875, -119.7588) (81.0129, -118.4743) (81.0887, -117.1447) (81.2394, -115.7626) (81.4789, -114.3687) (81.8013, -113.0103) (82.1793, -111.7216) (82.4671, -110.8931) (82.6087, -110.4853) knots 0 0 0 0 0.124973 0.252876 0.385371 0.524366 0.669742 0.809378 0.942972 1.072465 1.072465 1.072465 1.072465
  spline S9 degree 3 poles (82.6087, -105.7211) (82.5225, -105.7266) (82.3503, -105.7376) (82.0912, -105.7267) (81.8337, -105.6958) (81.5788, -105.6435) (81.3276, -105.5711) (81.0815, -105.4792) (80.8404, -105.3703) (80.6861, -105.2842) (80.6087, -105.241) knots 0 0 0 0 0.12386 0.247576 0.371585 0.495852 0.620749 0.746432 0.87277 1 1 1 1
  spline S10 degree 3 poles (80.6087, -105.241) (80.5366, -105.427) (80.3932, -105.7971) (80.0854, -106.5229) (79.6759, -107.4113) (79.1522, -108.4587) (78.79, -109.149) (78.6087, -109.4947) knots 0 0 0 0 0.127199 0.253182 0.502754 0.751027 1 1 1 1
  line L17 (88.5347, -92.0183) -> (64.5347, -92.0183)
  line L18 (86.0187, 21.9426) -> (67.0507, 21.9426)
  line L19 (86.5054, 21.5572) -> (66.564, 21.5572)
  spline S11 degree 3 poles (65.5507, 2.9586) (65.6964, 3.1577) (65.9904, 3.5593) (66.6379, 4.3327) (67.317, 5.0919) (67.9632, 5.8885) (68.3325, 6.4173) (68.5938, 6.864) (68.7698, 7.2138) (68.9262, 7.5783) (69.009, 7.8311) (69.0507, 7.9586) knots 0 0 0 0 0.074013 0.149267 0.302447 0.379596 0.456855 0.495662 0.534746 0.574288 0.614507 0.614507 0.614507 0.614507
  spline S12 degree 3 poles (87.5187, 2.9586) (87.3729, 3.1577) (87.079, 3.5593) (86.4315, 4.3327) (85.7524, 5.0919) (85.1062, 5.8885) (84.7369, 6.4173) (84.4756, 6.864) (84.2995, 7.2138) (84.1432, 7.5783) (84.0604, 7.8311) (84.0187, 7.9586) knots 0 0 0 0 0.074013 0.149267 0.302447 0.379596 0.456855 0.495662 0.534746 0.574288 0.614507 0.614507 0.614507 0.614507
  spline S13 degree 3 poles (64.0347, -2.0414) (64.0378, -1.8186) (64.0441, -1.3733) (64.1036, -0.7087) (64.2091, -0.0528) (64.3687, 0.5892) (64.5832, 1.2135) (64.854, 1.8174) (65.175, 2.4024) (65.4249, 2.7724) (65.5507, 2.9586) knots 0 0 0 0 0.066832 0.133581 0.19996 0.265954 0.331772 0.397749 0.464268 0.531651 0.531651 0.531651 0.531651
  spline S14 degree 3 poles (89.0347, -2.0414) (89.0315, -1.8186) (89.0253, -1.3733) (88.9658, -0.7087) (88.8602, -0.0528) (88.7007, 0.5892) (88.4861, 1.2135) (88.2154, 1.8174) (87.8944, 2.4024) (87.6445, 2.7724) (87.5187, 2.9586) knots 0 0 0 0 0.066832 0.133581 0.19996 0.265954 0.331772 0.397749 0.464268 0.531651 0.531651 0.531651 0.531651
  arc A0 (86.5054, 21.5572) -> (86.0187, 21.9426) centre (86.0187, 21.4426) ccw
  arc A1 (67.0507, 21.9426) -> (66.564, 21.5572) centre (67.0507, 21.4426) ccw
  spline S15 degree 3 poles (69.0507, 7.9586) (69.1048, 8.1594) (69.2156, 8.5706) (69.3, 9.2224) (69.3274, 9.9149) (69.2899, 10.6501) (69.1935, 11.4267) (69.0418, 12.2434) (68.8389, 13.0972) (68.5053, 14.3035) (68.0092, 15.8616) (67.385, 17.7579) (66.9256, 19.3605) (66.6574, 20.6296) (66.5946, 21.2529) (66.564, 21.5572) knots 0 0 0 0 0.062347 0.127633 0.196641 0.270049 0.348203 0.431234 0.519115 0.611423 0.806629 1.009594 1.210352 1.306485 1.398176 1.398176 1.398176 1.398176
  spline S16 degree 3 poles (84.0187, 7.9586) (83.9646, 8.1594) (83.8537, 8.5706) (83.7694, 9.2224) (83.7419, 9.9149) (83.7795, 10.6501) (83.8758, 11.4267) (84.0275, 12.2434) (84.2305, 13.0972) (84.5641, 14.3035) (85.0602, 15.8616) (85.6844, 17.7579) (86.1438, 19.3605) (86.412, 20.6296) (86.4747, 21.2529) (86.5054, 21.5572) knots 0 0 0 0 0.062347 0.127633 0.196641 0.270049 0.348203 0.431234 0.519115 0.611423 0.806629 1.009594 1.210352 1.306485 1.398176 1.398176 1.398176 1.398176
  line L20 (87.5347, 22.9586) -> (65.5347, 22.9586)
  spline S17 degree 3 poles (68.0347, 7.9586) (67.9341, 7.7425) (67.7309, 7.3057) (67.356, 6.6759) (66.9479, 6.0446) (66.507, 5.4116) (66.0373, 4.7821) (65.376, 3.965) (64.8704, 3.3602) (64.5347, 2.9586) knots 0 0 0 0 0.071451 0.144434 0.219638 0.296973 0.375788 0.45523 0.612272 0.612272 0.612272 0.612272
  spline S18 degree 3 poles (85.0347, 7.9586) (85.1352, 7.7425) (85.3385, 7.3057) (85.7134, 6.6759) (86.1215, 6.0446) (86.5624, 5.4116) (87.0321, 4.7821) (87.6933, 3.965) (88.1989, 3.3602) (88.5347, 2.9586) knots 0 0 0 0 0.071451 0.144434 0.219638 0.296973 0.375788 0.45523 0.612272 0.612272 0.612272 0.612272
  spline S19 degree 3 poles (64.5347, 2.9586) (64.3911, 2.7739) (64.1774, 2.4991) (63.9218, 2.1157) (63.748, 1.8257) (63.5925, 1.5302) (63.456, 1.229) (63.3397, 0.9215) (63.2434, 0.608) (63.1661, 0.2888) (63.0876, -0.1452) (63.032, -0.6991) (63.0156, -1.3692) (63.0177, -1.8174) (63.0187, -2.0414) knots 0 0 0 0 0.070131 0.104405 0.138173 0.17151 0.20452 0.237328 0.270066 0.302853 0.33579 0.402309 0.469592 0.53679 0.53679 0.53679 0.53679
  spline S20 degree 3 poles (88.5347, 2.9586) (88.6782, 2.7739) (88.8919, 2.4991) (89.1476, 2.1157) (89.3214, 1.8257) (89.4769, 1.5302) (89.6133, 1.229) (89.7297, 0.9215) (89.826, 0.608) (89.9033, 0.2888) (89.9818, -0.1452) (90.0373, -0.6991) (90.0538, -1.3692) (90.0517, -1.8174) (90.0507, -2.0414) knots 0 0 0 0 0.070131 0.104405 0.138173 0.17151 0.20452 0.237328 0.270066 0.302853 0.33579 0.402309 0.469592 0.53679 0.53679 0.53679 0.53679
  spline S21 degree 3 poles (65.5347, 21.9426) (65.5515, 21.6255) (65.587, 20.9582) (65.7998, 19.9366) (66.0794, 18.863) (66.5301, 17.4009) (67.0229, 15.9594) (67.4927, 14.5516) (67.8052, 13.5646) (68.0668, 12.6387) (68.2684, 11.7806) (68.4046, 10.9927) (68.4681, 10.2734) (68.4582, 9.6188) (68.3794, 9.0215) (68.239, 8.4702) (68.1022, 8.1275) (68.0347, 7.9586) knots 0 0 0 0 0.095122 0.200216 0.312183 0.428034 0.659064 0.769198 0.873257 0.96964 1.057768 1.137592 1.209313 1.274064 1.333591 1.389675 1.444205 1.444205 1.444205 1.444205
  spline S22 degree 3 poles (87.5347, 21.9426) (87.5178, 21.6255) (87.4824, 20.9582) (87.2696, 19.9366) (86.99, 18.863) (86.5393, 17.4009) (86.0465, 15.9594) (85.5767, 14.5516) (85.2642, 13.5646) (85.0026, 12.6387) (84.801, 11.7806) (84.6648, 10.9927) (84.6013, 10.2734) (84.6112, 9.6188) (84.69, 9.0215) (84.8303, 8.4702) (84.9672, 8.1275) (85.0347, 7.9586) knots 0 0 0 0 0.095122 0.200216 0.312183 0.428034 0.659064 0.769198 0.873257 0.96964 1.057768 1.137592 1.209313 1.274064 1.333591 1.389675 1.444205 1.444205 1.444205 1.444205
  line L21 (65.5347, 21.9426) -> (65.5347, 22.9586)
  line L22 (87.5347, 21.9426) -> (87.5347, 22.9586)
  line L23 (84.5347, -121.0183) -> (81.6078, -121.0183)
  line L24 (79.3547, -121.0183) -> (68.6542, -121.0183)
  spline S23 degree 3 poles (63.5187, -96.0183) (63.5195, -96.8706) (63.5207, -98.1467) (63.6215, -99.8428) (63.7599, -101.1043) (63.97, -102.3559) (64.2564, -103.5957) (64.6116, -104.825) (64.8973, -105.6314) (65.0407, -106.0362) knots 0 0 0 0 0.25561 0.382747 0.509496 0.636178 0.763224 0.891032 1.019834 1.019834 1.019834 1.019834
  spline S24 degree 3 poles (89.5507, -96.0183) (89.5461, -97.0883) (89.5393, -98.6901) (89.3558, -100.8155) (89.0973, -102.3908) (88.7203, -103.947) (88.0781, -106.0086) (87.0427, -108.5183) (86.0072, -111.028) (85.365, -113.0896) (84.9881, -114.6459) (84.7295, -116.2211) (84.546, -118.3466) (84.5392, -119.9483) (84.5347, -121.0183) knots 0 0 0 0 0.320849 0.480281 0.639462 0.799243 0.960292 1.286737 1.613182 1.774231 1.934012 2.093192 2.252625 2.573474 2.573474 2.573474 2.573474
  line L25 (81.5347, -92.0183) -> (81.5347, -121.0183)
  line L26 (71.5347, -92.0183) -> (71.5347, -121.0183)
  line L27 (81.4977, -92.0183) -> (81.4977, -94.5183)
  line L28 (79.7197, -92.0183) -> (79.7197, -94.5183)
  line L29 (82.2437, -92.0183) -> (82.2437, -94.5183)
  line L30 (80.4657, -92.0183) -> (80.4657, -94.5183)
  line L31 (67.9297, -92.0183) -> (67.9297, -94.5183)
  line L32 (66.1517, -92.0183) -> (66.1517, -94.5183)
  line L33 (64.5347, -92.0183) -> (64.5347, -32.0183)
  line L34 (88.5347, -92.0183) -> (88.5347, -32.0183)
  line L35 (63.5187, -96.0183) -> (63.5187, -32.0183)
  line L36 (89.5507, -96.0183) -> (89.5507, -32.0183)
  spline S25 degree 3 poles (64.5347, -32.0183) (64.5343, -31.8095) (64.5337, -31.3924) (64.4957, -30.7671) (64.4088, -30.1457) (64.2847, -29.5299) (64.1606, -28.914) (64.0737, -28.2927) (64.0357, -27.6674) (64.035, -27.2502) (64.0347, -27.0414) knots 0 0 0 0 0.062631 0.12514 0.187761 0.250672 0.313584 0.376205 0.438713 0.501345 0.501345 0.501345 0.501345
  spline S26 degree 3 poles (88.5347, -32.0183) (88.535, -31.8095) (88.5357, -31.3924) (88.5737, -30.7671) (88.6606, -30.1457) (88.7847, -29.5299) (88.9088, -28.914) (88.9957, -28.2927) (89.0337, -27.6674) (89.0343, -27.2502) (89.0347, -27.0414) knots 0 0 0 0 0.062631 0.12514 0.187761 0.250672 0.313584 0.376205 0.438713 0.501345 0.501345 0.501345 0.501345
  spline S27 degree 3 poles (63.0187, -27.0414) (63.019, -27.2502) (63.0197, -27.6674) (63.0577, -28.2927) (63.1446, -28.914) (63.2687, -29.5299) (63.3928, -30.1457) (63.4797, -30.7671) (63.5177, -31.3924) (63.5183, -31.8095) (63.5187, -32.0183) knots 0 0 0 0 0.062631 0.12514 0.187761 0.250672 0.313584 0.376205 0.438713 0.501345 0.501345 0.501345 0.501345
  spline S28 degree 3 poles (90.0507, -27.0414) (90.0503, -27.2502) (90.0497, -27.6674) (90.0117, -28.2927) (89.9248, -28.914) (89.8007, -29.5299) (89.6766, -30.1457) (89.5897, -30.7671) (89.5517, -31.3924) (89.551, -31.8095) (89.5507, -32.0183) knots 0 0 0 0 0.062631 0.12514 0.187761 0.250672 0.313584 0.376205 0.438713 0.501345 0.501345 0.501345 0.501345
  line L37 (64.0347, -27.0414) -> (64.0347, -2.0414)
  line L38 (89.0347, -27.0414) -> (89.0347, -2.0414)
  line L39 (63.0187, -27.0414) -> (63.0187, -2.0414)
  line L40 (90.0507, -27.0414) -> (90.0507, -2.0414)
  line L41 (-90.4666, -35.917) -> (-90.4421, -35.912)
  ellipse E0 centre (-90.3436, -35.8942) end of major axis (-89.5599, -35.7336) minor radius 0.0024 (-90.1871, -35.8598) -> (-90.4421, -35.912) ccw
  ellipse E1 centre (-90.3436, -35.8942) end of major axis (-89.5599, -35.7336) minor radius 0.0024 (-89.5599, -35.7336) -> (-90.012, -35.8241) ccw
  line L42 (-89.5598, -35.7343) -> (-89.5599, -35.7336)
  ellipse E2 centre (-103.6595, -35.8942) end of major axis (-104.4432, -35.7336) minor radius 0.0024 (-103.9925, -35.8238) -> (-104.4432, -35.7336) ccw
  line L43 (-102.6465, -36.0989) -> (-102.414, -36.1464)
  line L44 (-104.4433, -35.7343) -> (-104.4432, -35.7336)
  ellipse E3 centre (-90.876, -36.0379) end of major axis (-90.1179, -35.7824) minor radius 0.0023 (-90.8075, -36.0125) -> (-90.959, -36.0635) ccw
  ellipse E4 centre (-90.876, -36.0379) end of major axis (-90.1179, -35.7824) minor radius 0.0023 (-90.6893, -35.9727) -> (-90.8017, -36.0105) ccw
  ellipse E5 centre (-90.876, -36.0379) end of major axis (-90.1179, -35.7824) minor radius 0.0023 (-90.1179, -35.7824) -> (-90.2894, -35.8387) ccw
  line L45 (-90.1151, -35.7905) -> (-90.1179, -35.7824)
  line L46 (-92.6745, -35.892) -> (-94.3279, -30.9862)
  ellipse E6 centre (-88.2336, -36.9513) end of major axis (-89.011, -37.1401) minor radius 0.1369 (-88.5284, -36.8904) -> (-88.5454, -36.8957) ccw
  line L47 (-88.8161, -36.9626) -> (-88.6256, -36.9123)
  ellipse E7 centre (-88.0011, -37.9088) end of major axis (-88.487, -38.0267) minor radius 0.0856 (-88.1215, -37.8518) -> (-88.268, -38.0451) ccw
  ellipse E8 centre (-106.692, -35.8675) end of major axis (-107.4918, -35.8877) minor radius 0.1339 (-107.0433, -35.7558) -> (-107.4918, -35.8877) ccw
  line L48 (-106.7191, -35.7343) -> (-105.1456, -35.6869)
  line L49 (-105.1456, -35.6869) -> (-105.1407, -35.8842)
  ellipse E9 centre (-106.6424, -37.8387) end of major axis (-107.4421, -37.8589) minor radius 0.1339 (-106.3704, -37.7061) -> (-106.6695, -37.7055) ccw
  line L50 (-105.1456, -35.6869) -> (-105.1556, -35.2934)
  line L51 (-105.1726, -34.6185) -> (-105.1969, -33.6529)
  ellipse E10 centre (-107.0372, -22.1681) end of major axis (-109.1266, -22.2207) minor radius 0.3499 (-107.8913, -21.8696) -> (-108.146, -21.8986) ccw
  ellipse E11 centre (-107.0149, -23.0551) end of major axis (-109.1042, -23.1077) minor radius 0.3499 (-107.8776, -22.7574) -> (-108.1131, -22.7842) ccw
  ellipse E12 centre (-107.0149, -23.0551) end of major axis (-108.5144, -23.0929) minor radius 0.2511 (-106.2212, -22.8225) -> (-108.4706, -23.151) ccw
  ellipse E13 centre (-106.6424, -37.8387) end of major axis (-107.1422, -37.8513) minor radius 0.0837 (-106.7161, -37.7577) -> (-106.8908, -37.9174) ccw
  ellipse E14 centre (-104.2402, -35.8143) end of major axis (-105.0382, -35.7571) minor radius 0.0023 (-104.3543, -35.8038) -> (-105.0382, -35.7571) ccw
  line L52 (-104.3543, -35.8038) -> (-104.2957, -35.808)
  line L53 (-104.0591, -35.8248) -> (-102.7996, -35.9144)
  line L54 (-102.7996, -35.9144) -> (-102.8149, -36.128)
  line L55 (-105.0391, -35.7703) -> (-105.0382, -35.7571)
  line L56 (-102.7996, -35.9144) -> (-102.6804, -34.2494)
  line L57 (-90.8802, -35.4793) -> (-90.8125, -35.8215)
  line L58 (-91.8484, -36.3028) -> (-90.3751, -36.0314)
  ellipse E15 centre (-90.3078, -35.9204) end of major axis (-89.523, -35.765) minor radius 0.0964 (-90.3751, -36.0314) -> (-89.6659, -35.7386) ccw
  line L59 (-89.6659, -35.7386) -> (-90.1877, -35.7476)
  line L60 (-89.5215, -35.7727) -> (-89.523, -35.765)
  line L61 (-88.3661, -35.5973) -> (-88.3552, -35.7011)
  line L62 (-88.8717, -35.905) -> (-87.9961, -35.8084)
  ellipse E16 centre (-87.8896, -35.8313) end of major axis (-87.0939, -35.748) minor radius 0.0342 (-87.1292, -35.7417) -> (-87.9961, -35.8084) ccw
  ellipse E17 centre (-89.3359, -22.0195) end of major axis (-87.2573, -21.8018) minor radius 0.0893 (-87.3996, -21.7845) -> (-87.9008, -21.8045) ccw
  ellipse E18 centre (-89.2423, -22.9138) end of major axis (-87.1636, -22.6961) minor radius 0.0893 (-87.3086, -22.6787) -> (-87.376, -22.6792) ccw
  ellipse E19 centre (-87.6815, -37.8186) end of major axis (-88.1788, -37.8707) minor radius 0.0214 (-88.058, -37.8439) -> (-88.1554, -37.8616) ccw
  ellipse E20 centre (-87.6815, -37.8186) end of major axis (-87.1842, -37.7665) minor radius 0.0214 (-87.2241, -37.7624) -> (-87.4937, -37.7791) ccw
  ellipse E21 centre (-100.3016, -37.1544) end of major axis (-99.5954, -37.3004) minor radius 0.4312 (-101.0098, -37.1038) -> (-100.9931, -37.1669) ccw
  line L63 (-104.6977, -35.2091) -> (-104.7563, -35.7688)
  ellipse E22 centre (-106.1135, -35.8313) end of major axis (-105.3178, -35.9146) minor radius 0.0342 (-106.1441, -35.7937) -> (-106.8469, -35.7413) ccw
  line L64 (-106.1441, -35.7937) -> (-105.131, -35.898)
  line L65 (-104.5611, -35.7849) -> (-104.5019, -35.2196)
  ellipse E23 centre (-104.6672, -22.0195) end of major axis (-106.7458, -21.8018) minor radius 0.0893 (-106.1023, -21.8045) -> (-106.6035, -21.7845) ccw
  ellipse E24 centre (-104.7608, -22.9138) end of major axis (-106.8394, -22.6961) minor radius 0.0893 (-106.627, -22.6792) -> (-106.6944, -22.6787) ccw
  ellipse E25 centre (-104.7608, -22.9138) end of major axis (-106.2526, -22.7576) minor radius 0.0641 (-106.2124, -22.7472) -> (-106.2158, -22.776) ccw
  ellipse E26 centre (-106.3216, -37.8186) end of major axis (-105.8243, -37.8707) minor radius 0.0214 (-105.8552, -37.8748) -> (-105.9451, -37.8439) ccw
  ellipse E27 centre (-106.3216, -37.8186) end of major axis (-106.8189, -37.7665) minor radius 0.0214 (-106.5094, -37.7791) -> (-106.7876, -37.7774) ccw
  line L66 (-101.826, -33.1767) -> (-102.4257, -36.2056)
  line L67 (-104.13, -35.7528) -> (-104.208, -35.746)
  ellipse E28 centre (-103.6953, -35.9204) end of major axis (-104.4801, -35.765) minor radius 0.0964 (-104.208, -35.746) -> (-103.8203, -35.993) ccw
  line L68 (-103.8203, -35.993) -> (-102.2947, -36.3213)
  line L69 (-102.2947, -36.3213) -> (-102.3039, -36.3677)
  line L70 (-104.4816, -35.7727) -> (-104.4801, -35.765)
  line L71 (-102.3501, -36.286) -> (-102.2947, -36.3213)
  line L72 (-102.2947, -36.3213) -> (-101.6756, -33.1943)
  line L73 (-90.0124, -35.8299) -> (-89.8444, -35.8178)
  ellipse E29 centre (-89.7629, -35.8143) end of major axis (-88.9649, -35.7571) minor radius 0.0023 (-88.9649, -35.7571) -> (-89.8444, -35.8178) ccw
  line L74 (-88.964, -35.7703) -> (-88.9649, -35.7571)
  line L75 (-91.6081, -33.1212) -> (-91.6089, -33.1103)
  line L76 (-87.7345, -35.5276) -> (-87.7394, -35.7201)
  line L77 (-88.9524, -35.7305) -> (-87.4217, -35.7322)
  ellipse E30 centre (-87.311, -35.8675) end of major axis (-86.5113, -35.8877) minor radius 0.1339 (-86.5113, -35.8877) -> (-87.4217, -35.7322) ccw
  ellipse E31 centre (-86.9659, -22.1681) end of major axis (-89.0552, -22.1154) minor radius 0.3499 (-85.857, -21.8986) -> (-86.1118, -21.8696) ccw
  ellipse E32 centre (-86.9882, -23.0551) end of major axis (-89.0775, -23.0024) minor radius 0.3499 (-85.89, -22.7842) -> (-86.1255, -22.7574) ccw